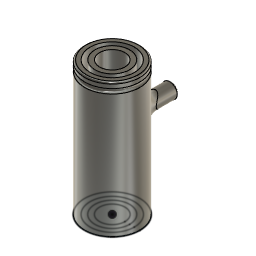
NoiseMakerSimple (Autodesk Fusion 360 design; units mm, degrees)
Autodesk Fusion 360 part; units mm, degrees
sketch "Sketch1" plane through (0, 0, 0) normal (0, 0, 1) x (1, 0, 0)
  circle A0 centre (0, 0) radius 17.5
  circle A1 centre (0, 0) radius 14
  circle A2 centre (0, 0) radius 11
  circle A3 centre (0, 0) radius 8
  dimension "d2" = 35
  dimension "d3" = 28
  dimension "d4" = 22
  dimension "d5" = 16
  constraint coincident A0.centre A1.centre
  constraint concentric A0 A1
  constraint concentric A1 A2
  constraint concentric A0 A3
  measures "d2" diameter of A0
  measures "d3" diameter of A1
  measures "d4" diameter of A2
  measures "d5" diameter of A3
extrude "Extrude1" add sketch "Sketch1" along normal blind 85 contours A0 makes body 1
extrude "Extrude2" add sketch "Sketch1" along normal blind 85 separate body contours A2 makes body 2
extrude "Extrude3" add sketch "Sketch1" along normal blind 3.5 contours A0 | A1 | A2 bodies 1 2
sketch "Sketch2" plane through (0, 0, 0) normal (0, 1, 0) x (1, 0, 0)
  circle A0 centre (0, -50) radius 4.75
  line L0 (-17.5, -85) -> (17.5, -85)
  circle A1 centre (0, -50) radius 3.25
  dimension "d13" = 9.5
  dimension "d14" = 35
  dimension "d15" = 6.5
  constraint concentric A0 A1
  measures "d13" diameter of A0
  measures "d14" distance of A0.centre L0
  measures "d15" diameter of A1
extrude "Extrude4" add sketch "Sketch2" along normal blind 37.5 separate body makes body 3
extrude "Extrude5" add sketch "Sketch1" along normal blind 85 separate body contours A1 | A2 | A3 makes body 4
combine "Combine1" operation cut target body 3 tool bodies 4
sketch "Sketch3" plane through (0, 37.5, 0) normal (0, 1, 0) x (-1, 0, 0)
  circle A0 centre (0, 50) radius 3.25
  circle A1 centre (0, 50) radius 4.75
  circle A2 centre (0, 50) radius 3.25
  constraint concentric A0 A2
extrude "Extrude6" cut sketch "Sketch3" against normal blind 26 contours A0 A2 bodies 1
combine "Combine2" operation add target body 3 tool bodies 1
fillet "Fillet1" radius 10 1 edges at (4.75, 16.843, 50) on bodies 3
fillet "Fillet2" radius 1 1 edges at (-4.4286, 37.5, 51.7177) on bodies 3
sketch "Sketch4" plane through (0, 0, 0) normal (0, 1, 0) x (1, 0, 0)
  circle A0 centre (-17.4, -80) radius 1.5
  line L0 (-17.5, -85) -> (17.5, -85)
  dimension "d26" = 3
  dimension "d27" = 5
  dimension "d28" = 0.1
  measures "d26" diameter of A0
  measures "d27" distance of A0.centre L0
  measures "d28" horizontal distance of A0.centre L0.start
revolve "Revolve1" cut sketch "Sketch4" angle 360 about axis through (0, 0, 0) along (0, 0, -1) bodies 3
fillet "Fillet3" radius 1 1 edges at (-16.3157, -6.3283, 85) on bodies 3
equation "ExternalDiam = 35 mm"
equation "d2 = ExternalDiam"
equation "d3 = ExternalDiam - 7 mm"
equation "d4 = ExternalDiam - 7 mm - 6 mm"
equation "d5 = ExternalDiam - 7 mm - 6 mm - 6 mm"
equation "OverallLength = 85 mm"
equation "d7 = OverallLength"
equation "d9 = OverallLength"
equation "d16 = ExternalDiam / 2 + 20 mm"
equation "d18 = OverallLength"
